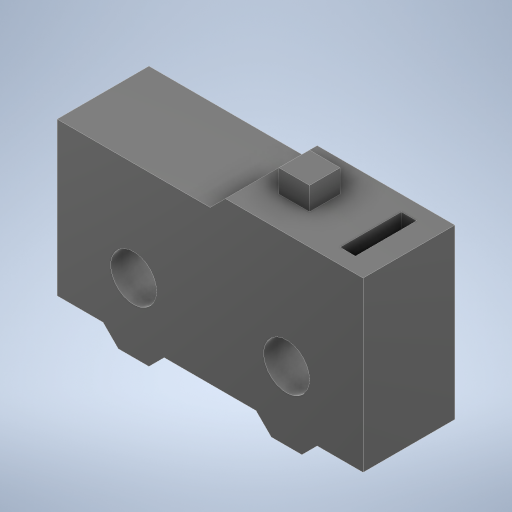
# Autodesk Inventor part: Limit switch body
Saved by Autodesk Inventor 2023 (Build 270158000, 158)
## iProperties
Created: 2023-12-14
Part Number: Limit switch body
Material: Generic
Document SubType Name: Modeling
Designer: User
Density: 1 g/cm^3
Appearance: Smooth - Black
Author: User
Autodesk Inventor part; units mm, degrees
ref_plane "YZ Plane" through (0, 0, 0) normal (1, 0, 0) x (0, 1, 0)
ref_plane "XZ Plane" through (0, 0, 0) normal (0, 1, 0) x (-1, 0, 0)
ref_plane "XY Plane" through (0, 0, 0) normal (0, 0, 1) x (1, 0, 0)
sketch "Sketch1" plane through (0, 0, 0) normal (0, 0, 1) x (1, 0, 0)
  line L0 (0, 0) -> (20, 0)
  line L1 (20, 0) -> (20, -10)
  line L2 (20, -10) -> (0, -10)
  line L3 (0, -10) -> (0, 0)
  dimension "d0" = 20
  dimension "d1" = 10
  constraints: 8 end point, 2 parallel, 1 horizontal, 1 perpendicular
  measures "d0" distance of L1.end L2.end
  measures "d1" distance of L0.end L1.end
extrude "Extrusion1" add sketch "Sketch1" along normal blind 6
sketch "Sketch2" plane through (0, 0, 0) normal (0, 1, 0) x (1, 0, 0)
  line L0 (20, 0) -> (20, -6) projected
  line L1 (20, 0) -> (10, 0)
  line L2 (10, 0) -> (10, -6)
  line L3 (10, -6) -> (20, -6)
  line L4 (20, -6) -> (20, 0)
  point P0 (0, 0)
  dimension "d4" = 10
  constraints: 8 end point, 2 parallel, 1 horizontal, 1 perpendicular
  measures "d4" distance of L3.end L2.end
extrude "Extrusion2" add sketch "Sketch2" along normal blind 1
chamfer "Chamfer2" distance 1 angle 45 1 edges at (10, 1, 3)
sketch "Sketch3" plane through (0, -10, 0) normal (0, -1, 0) x (1, 0, 0)
  line L0 (0, 6) -> (3, 6) construction
  line L1 (3, 6) -> (3, 0) construction
  line L2 (3, 0) -> (0, 0) construction
  line L3 (0, 0) -> (0, 6) construction
  line L4 (3, 6) -> (7, 6)
  line L5 (7, 6) -> (7, 0)
  line L6 (7, 0) -> (3, 0)
  line L7 (3, 0) -> (3, 6)
  line L8 (7, 6) -> (13, 6) construction
  line L9 (13, 6) -> (13, 0) construction
  line L10 (13, 0) -> (7, 0) construction
  line L11 (7, 0) -> (7, 6) construction
  line L12 (13, 6) -> (17, 6)
  line L13 (17, 6) -> (17, 0)
  line L14 (17, 0) -> (13, 0)
  line L15 (13, 0) -> (13, 6)
  dimension "d13" = 3
  dimension "d14" = 4
  dimension "d15" = 6
  dimension "d16" = 4
  constraints: 32 end point, 8 parallel, 4 horizontal, 4 perpendicular
  measures "d13" distance of L1.end L2.end
  measures "d14" distance of L5.end L6.end
  measures "d15" distance of L9.end L10.end
  measures "d16" distance of L13.end L14.end
extrude "Extrusion3" add sketch "Sketch3" along normal blind 1
chamfer "Chamfer3" distance 1 angle 45 4 edges at (3, -11, 3) (7, -11, 3) (13, -11, 3) (17, -11, 3)
sketch "Sketch4" plane through (0, -10, 0) normal (0, -1, 0) x (1, 0, 0)
  line L0 (0, 6) -> (2.9323, 6) construction
  line L1 (0, 5) -> (2.9323, 5) construction
  line L2 (0, 0) -> (2.9323, 0) construction
  line L3 (2.9323, 1) -> (1, 1) construction
  line L4 (1, 1) -> (1, 5) construction
  line L5 (1, 5) -> (2.9323, 5) construction
  line L6 (2, 5) -> (2, 1) construction
  line L7 (1, 5) -> (2, 5)
  line L8 (2, 5) -> (2, 1)
  line L9 (2, 1) -> (1, 1)
  line L10 (1, 1) -> (1, 5)
  dimension "d22" = 1
  dimension "d23" = 1
  dimension "d24" = 1
  constraints: 22 end point, 3 parallel, 2 point on line, 1 horizontal, 1 perpendicular
  measures "d22" distance between parallel lines of L0 L1
  measures "d23" distance between parallel lines of L2 L3
  measures "d24" distance between parallel lines of L4 L6
extrude "Extrusion4" cut sketch "Sketch4" against normal blind 1
sketch "Sketch5" plane through (7, -10, 0) normal (0, -1, 0) x (1, 0, 0)
  line L0 (0, 0.2008) -> (0, 5.4827) construction
  line L1 (3, 0.2008) -> (3, 5.4827) construction
  line L2 (4, 0.2008) -> (4, 5.4827) construction
  line L3 (6, 0) -> (0.2208, 0) construction
  line L4 (6, 1) -> (0.2208, 1) construction
  line L5 (6, 6) -> (0.5976, 6) construction
  line L6 (6, 5) -> (0.5976, 5) construction
  line L7 (4, 1) -> (3, 1)
  line L8 (3, 1) -> (3, 5)
  line L9 (3, 5) -> (4, 5)
  line L10 (4, 5) -> (4, 1)
  point P0 (-7, 0)
  dimension "d27" = 3
  dimension "d28" = 1
  dimension "d29" = 1
  dimension "d30" = 1
  constraints: 22 end point, 6 parallel, 2 point on line, 1 horizontal, 1 perpendicular
  measures "d27" distance between parallel lines of L0 L1
  measures "d28" distance between parallel lines of L1 L2
  measures "d29" distance between parallel lines of L3 L4
  measures "d30" distance between parallel lines of L5 L6
extrude "Extrusion5" cut sketch "Sketch5" against normal blind 1
sketch "Sketch6" plane through (20, -10, 0) normal (0, -1, 0) x (1, 0, 0)
  line L0 (0, 0) -> (0, 5.7185) construction
  line L1 (-1, 0) -> (-1, 5.7185) construction
  line L2 (-2, 0) -> (-2, 5.7185) construction
  line L3 (-0.3844, 0) -> (-2.7356, 0) construction
  line L4 (-0.3844, 1) -> (-2.7356, 1) construction
  line L5 (-0.4485, 6) -> (-2.495, 6) construction
  line L6 (-0.4485, 5) -> (-2.495, 5) construction
  line L7 (-1, 1) -> (-2, 1)
  line L8 (-2, 1) -> (-2, 5)
  line L9 (-2, 5) -> (-1, 5)
  line L10 (-1, 5) -> (-1, 1)
  point P0 (-20, 0)
  dimension "d33" = 1
  dimension "d34" = 1
  dimension "d35" = 1
  dimension "d36" = 1
  constraints: 22 end point, 6 parallel, 4 point on line, 1 horizontal, 1 perpendicular
  measures "d33" distance between parallel lines of L0 L1
  measures "d34" distance between parallel lines of L1 L2
  measures "d35" distance between parallel lines of L3 L4
  measures "d36" distance between parallel lines of L5 L6
extrude "Extrusion6" cut sketch "Sketch6" against normal blind 1
sketch "Sketch7" plane through (0, 1, 0) normal (0, 1, 0) x (1, 0, 0)
  line L0 (11, -5.3093) -> (11, -0.576) construction
  line L1 (12.5, -5.3093) -> (12.5, -0.576) construction
  line L2 (14.5, -5.3093) -> (14.5, -0.576) construction
  line L3 (15, 0) -> (12.0712, 0) construction
  line L4 (15, -2) -> (12.0712, -2) construction
  line L5 (15, -4) -> (12.0712, -4) construction
  line L6 (14.5, -4) -> (12.5, -4)
  line L7 (12.5, -4) -> (12.5, -2)
  line L8 (12.5, -2) -> (14.5, -2)
  line L9 (14.5, -2) -> (14.5, -4)
  point P0 (0, 0)
  dimension "d39" = 1.5
  dimension "d40" = 2
  dimension "d41" = 2
  dimension "d42" = 2
  constraints: 20 end point, 6 parallel, 4 point on line, 1 horizontal, 1 perpendicular
  measures "d39" distance between parallel lines of L0 L1
  measures "d40" distance between parallel lines of L1 L2
  measures "d41" distance between parallel lines of L3 L4
  measures "d42" distance between parallel lines of L4 L5
extrude "Extrusion7" add sketch "Sketch7" along normal blind 1.5
sketch "Sketch8" plane through (0, 1, 0) normal (0, 1, 0) x (1, 0, 0)
  line L0 (14.5, -5.3842) -> (14.5, -1) construction
  line L1 (17.5, -5.3842) -> (17.5, -1) construction
  line L2 (18.8144, -6) -> (15.3684, -6) construction
  line L3 (18.8144, -5) -> (14.5, -5) construction
  line L4 (18.8144, -1) -> (14.5, -1) construction
  line L5 (17.5, -5) -> (18.5, -5)
  line L6 (18.5, -5) -> (18.5, -1)
  line L7 (18.5, -1) -> (17.5, -1)
  line L8 (17.5, -1) -> (17.5, -5)
  point P0 (0, 0)
  dimension "d45" = 3
  dimension "d47" = 1
  dimension "d48" = 4
  dimension "d49" = 1
  constraints: 18 end point, 5 parallel, 5 point on line, 1 horizontal, 1 perpendicular, 1 vertical
  measures "d45" distance between parallel lines of L0 L1
  measures "d47" distance between parallel lines of L2 L3
  measures "d48" distance between parallel lines of L3 L4
  measures "d49" distance of L7.end L6.end
extrude "Extrusion8" cut sketch "Sketch8" against normal blind 1
sketch "Sketch9" plane through (0, 0, 0) normal (0, 0, -1) x (-1, 0, 0)
  line L0 (-20, -10) -> (-0.9385, -10) construction
  line L1 (-20, -6.5) -> (-0.9385, -6.5) construction
  line L2 (-13, -10) -> (-14, -11) construction
  line L3 (-13, -10) -> (-13, -3.6474) construction
  line L4 (-3, -10) -> (-3, -3.6474) construction
  line L5 (-5, -10) -> (-5, -3.6474) construction
  line L6 (-15, -10) -> (-15, -3.6474) construction
  circle A0 centre (-15, -6.5) radius 1.5
  circle A1 centre (-5, -6.5) radius 1.5
  point P0 (0, 0)
  dimension "d52" = 3.5
  dimension "d53" = 2
  dimension "d54" = 2
  dimension "d55" = 3
  dimension "d56" = 3
  constraints: 12 end point, 4 point on line, 3 parallel, 2 centre point, 2 vertical
  measures "d52" distance between parallel lines of L0 L1
  measures "d53" distance between parallel lines of L4 L5
  measures "d54" distance between parallel lines of L3 L6
  measures "d55" diameter of A0
  measures "d56" diameter of A1
extrude "Extrusion9" cut sketch "Sketch9" against normal blind 20
body "Solid1"
